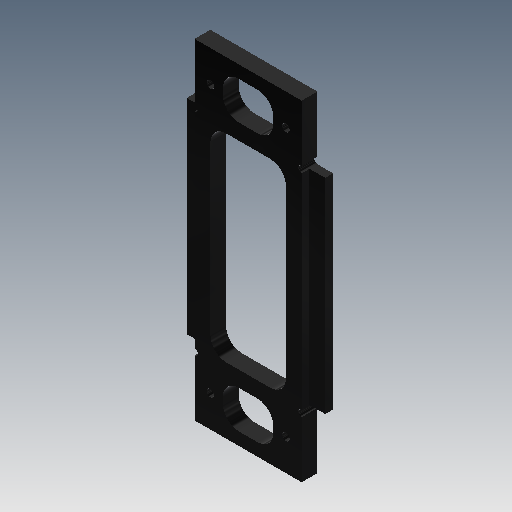
# Autodesk Inventor part: コックピット_2_サブフレーム_5
Saved by Autodesk Inventor 2017.3 (Build 213256000, 256)
## iProperties
Created: 2016-05-24
Part Number: コックピット_2_サブフレーム_5
Material: アセタール樹脂、黒
Document SubType Name: Modeling
Designer: hiroaki
Density: 1.425 g/cm^3
Appearance: 滑らか - 黒
Mass: 14.5233 g
Surface Area: 76.4272 cm^2
Volume: 10.1918 cm^3
Author: hiroaki
Autodesk Inventor part; units mm, degrees
ref_plane "YZ Plane" through (0, 0, 0) normal (1, 0, 0) x (0, 1, 0)
ref_plane "XZ Plane" through (0, 0, 0) normal (0, 1, 0) x (-1, 0, 0)
ref_plane "XY Plane" through (0, 0, 0) normal (0, 0, 1) x (1, 0, 0)
sketch "スケッチ1" plane through (0, 0, 0) normal (0, 0, 1) x (1, 0, 0)
  line L0 (-17, -52.5) -> (17, -52.5) construction
  line L1 (17, -52.5) -> (17, 52.5) construction
  line L2 (17, 52.5) -> (-17, 52.5) construction
  line L3 (-17, 52.5) -> (-17, -52.5) construction
  line L4 (-17, -52.5) -> (17, 52.5) construction
  line L5 (17, -52.5) -> (-17, 52.5) construction
  line L6 (-17, 34.6) -> (-17, 52.5)
  line L7 (-17, 52.5) -> (17, 52.5)
  line L8 (17, 52.5) -> (17, 34.6)
  line L9 (-17, -34.6) -> (-17, -52.5)
  line L10 (-17, -52.5) -> (17, -52.5)
  line L11 (17, -52.5) -> (17, -34.6)
  line L12 (-17, 32.5) -> (-22, 32.5)
  line L13 (-22, 32.5) -> (-22, -32.5)
  line L14 (-22, -32.5) -> (-17, -32.5)
  line L15 (17, 32.5) -> (22, 32.5)
  line L16 (22, 32.5) -> (22, -32.5)
  line L17 (22, -32.5) -> (17, -32.5)
  arc A0 (-17, 32.5) -> (-17, 34.6) centre (-17, 33.55) ccw
  arc A1 (-17, -34.6) -> (-17, -32.5) centre (-17, -33.55) ccw
  arc A2 (17, 34.6) -> (17, 32.5) centre (17, 33.55) ccw
  arc A3 (17, -32.5) -> (17, -34.6) centre (17, -33.55) ccw
  line L18 (0, 0) -> (17, 0) construction
  line L19 (0, 0) -> (0, 52.5) construction
  line L20 (-12, 42.5) -> (12, 42.5) construction
  line L21 (12, 42.5) -> (12, -42.5) construction
  line L22 (12, -42.5) -> (-12, -42.5) construction
  line L23 (-12, -42.5) -> (-12, 42.5) construction
  circle A4 centre (-12, 42.5) radius 1.2
  circle A5 centre (12, 42.5) radius 1.2
  circle A6 centre (12, -42.5) radius 1.2
  circle A7 centre (-12, -42.5) radius 1.2
  point P0 (0, 42.5)
  point P1 (0, 0)
  dimension "d87" = 1.05
  dimension "d88" = 105
  dimension "d89" = 5
  dimension "d90" = 20
  dimension "d91" = 34
  dimension "d92" = 2.4
  dimension "d93" = 5
  dimension "d94" = 10
  dimension "d95" = 10
  constraints: 48 end point, 10 vertical alignment, 9 perpendicular, 8 centre point, 8 point on circle, 6 midpoint, 5 equal radius, 5 horizontal, 4 coincident, 4 collinear, 4 parallel, 4 symmetric about line, 2 vertical, 1 tangent, 2 other
  measures "d87" radius of A0
  measures "d88" distance of L2.end L0.start
  measures "d89" distance between parallel lines of L13 L3
  measures "d90" distance between parallel lines of L2 L12
  measures "d91" distance of L1.end L2.end
  measures "d92" diameter of A4
  measures "d93" distance between parallel lines of L3 L23
  measures "d94" distance between parallel lines of L20 L2
  measures "d95" distance between parallel lines of L0 L22
extrude "押し出し1" add sketch "スケッチ1" along normal blind 5
sketch "スケッチ2" plane through (0, 0, 5) normal (0, 0, 1) x (1, 0, 0)
  line L0 (-17, 52.5) -> (-17, 34.6) projected
  line L1 (17, 34.6) -> (17, 52.5) projected
  line L2 (-40.5884, 60.19) -> (-17, 60.19)
  line L3 (-17, 60.19) -> (-17, -101.7483)
  line L4 (-17, -101.7483) -> (-40.5884, -101.7483)
  line L5 (-40.5884, -101.7483) -> (-40.5884, 60.19)
  line L6 (53.5752, 90.4043) -> (17, 90.4043)
  line L7 (17, 90.4043) -> (17, -93.5321)
  line L8 (17, -93.5321) -> (53.5752, -93.5321)
  line L9 (53.5752, -93.5321) -> (53.5752, 90.4043)
  point P0 (0, 0)
  constraints: 16 end point, 4 parallel, 2 collinear, 2 horizontal, 2 perpendicular
extrude "押し出し2" cut sketch "スケッチ2" against normal blind 2.5
sketch "スケッチ3" plane through (0, 0, 5) normal (0, 0, 1) x (1, 0, 0)
  line L0 (17, -32.5) -> (17, 32.5) projected
  line L1 (17, 52.5) -> (-17, 52.5) projected
  line L2 (-17, 32.5) -> (-17, -32.5) projected
  line L3 (-17, -52.5) -> (17, -52.5) projected
  circle A0 centre (-12, -42.5) radius 1.2 projected
  circle A1 centre (-12, 42.5) radius 1.2 projected
  line L4 (-8, -48.5) -> (8, -48.5)
  line L5 (8, -48.5) -> (8, -36.5)
  line L6 (8, -36.5) -> (-8, -36.5)
  line L7 (-8, -36.5) -> (-8, -48.5)
  line L8 (-12, -31.5) -> (12, -31.5)
  line L9 (12, -31.5) -> (12, 31.5)
  line L10 (12, 31.5) -> (-12, 31.5)
  line L11 (-12, 31.5) -> (-12, -31.5)
  line L12 (-8, 36.5) -> (8, 36.5)
  line L13 (8, 36.5) -> (8, 48.5)
  line L14 (8, 48.5) -> (-8, 48.5)
  line L15 (-8, 48.5) -> (-8, 36.5)
  line L16 (0, 52.5) -> (0, -52.5) construction
  line L17 (-17, 0) -> (17, 0) construction
  point P0 (0, 0)
  point P1 (0, -31.5)
  dimension "d100" = 4
  dimension "d101" = 4
  dimension "d102" = 4
  dimension "d103" = 4
  dimension "d104" = 6
  dimension "d105" = 5
  dimension "d106" = 6
  dimension "d107" = 5
  dimension "d108" = 5
  constraints: 28 end point, 6 parallel, 5 midpoint, 3 horizontal, 3 perpendicular, 1 point on line, 1 vertical alignment, 1 other
  measures "d100" distance between parallel lines of L3 L4
  measures "d101" distance from line of L7 A0.centre
  measures "d102" distance from line of A1.centre L15
  measures "d103" distance between parallel lines of L1 L14
  measures "d104" distance from line of L6 A0.centre
  measures "d105" distance between parallel lines of L8 L6
  measures "d106" distance from line of A1.centre L12
  measures "d107" distance between parallel lines of L10 L12
  measures "d108" distance between parallel lines of L2 L11
extrude "押し出し3" cut sketch "スケッチ3" against normal blind 10 contours L7 L6 L5 L4 | L11 L10 L9 L8 | L15 L14 L13 L12
fillet "フィレット1" radius 5 12 edges at (-8, 48.5, 2.5) (8, 48.5, 2.5) (-8, 36.5, 2.5) (8, 36.5, 2.5) (-12, 31.5, 2.5) (12, 31.5, 2.5) (12, -31.5, 2.5) (-12, -31.5, 2.5) (-8, -36.5, 2.5) (-8, -48.5, 2.5) (8, -48.5, 2.5) (8, -36.5, 2.5)
equation "\"d88\" = d83"
equation "\"d90\" = d84"
equation "\"d102\" = d101"
equation "\"d103\" = d100"
equation "\"d106\" = d104"
equation "\"d107\" = d105"
equation "\"d83\" = 105"
equation "\"d84\" = 20"
